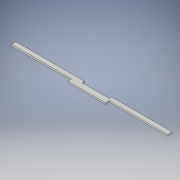
# Autodesk Inventor part: radialArmSawFence
Saved by Autodesk Inventor 2017 (Build 210142000, 142)
## iProperties
Created: 2018-08-06
Part Number: radialArmSawFence
Material: Generic
Document SubType Name: Modeling
Designer: Jake
Density: 1 g/cm^3
Appearance: Default
Author: Jake
Autodesk Inventor part; units mm, degrees
ref_plane "YZ Plane" through (0, 0, 0) normal (1, 0, 0) x (0, 1, 0)
ref_plane "XZ Plane" through (0, 0, 0) normal (0, 1, 0) x (-1, 0, 0)
ref_plane "XY Plane" through (0, 0, 0) normal (0, 0, 1) x (1, 0, 0)
sketch "Sketch1" plane through (0, 0, 0) normal (0, 1, 0) x (-1, 0, 0)
  line L0 (-942.975, -26.67) -> (-942.975, 26.67)
  line L1 (-942.975, 26.67) -> (-228.6, 26.67)
  line L2 (-228.6, 26.67) -> (-228.6, 71.12)
  line L3 (-228.6, 71.12) -> (228.6, 71.12)
  line L4 (228.6, 71.12) -> (228.6, 26.67)
  line L5 (228.6, 26.67) -> (962.025, 26.67)
  line L6 (962.025, 26.67) -> (962.025, -26.67)
  line L7 (962.025, -26.67) -> (124.46, -26.67)
  line L8 (124.46, -26.67) -> (124.46, 2.54)
  line L9 (124.46, 2.54) -> (-205.74, 2.54)
  line L10 (-205.74, 2.54) -> (-205.74, -26.67)
  line L11 (-205.74, -26.67) -> (-942.975, -26.67)
  point P0 (0, 0)
  point P1 (-942.975, 0)
  point P2 (0, 71.12)
  dimension "d0" = 1905
  dimension "d1" = 53.34
  dimension "d2" = 53.34
  dimension "d3" = 68.58
  dimension "d4" = 22.86
  dimension "d5" = 104.14
  dimension "d6" = 29.21
  dimension "d7" = 457.2
  dimension "d8" = 714.375
  constraints: 24 end point, 10 perpendicular, 2 midpoint, 1 horizontal, 1 horizontal alignment, 1 point on line, 1 vertical alignment
  measures "d0" distance between parallel lines of L0 L6
  measures "d1" distance between parallel lines of L5 L7
  measures "d2" distance of L0.start L0.end
  measures "d3" distance between parallel lines of L3 L9
  measures "d4" distance between parallel lines of L2 L10
  measures "d5" distance between parallel lines of L4 L8
  measures "d6" distance of L9.end L10.end
  measures "d7" distance of L2.end L3.end
  measures "d8" distance of L0.end L1.end
extrude "Extrusion1" add sketch "Sketch1" along normal blind 19.05
equation "\"d2\" = d1"
body "Solid1"
